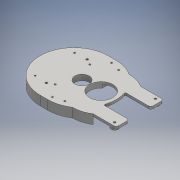
# Autodesk Inventor part: AZ-FLDIC-FWup top adapter
Saved by Autodesk Inventor 2016 (Build 200138000, 138)
## iProperties
Created: 2015-08-14
Part Number: AZ-FLDIC-FWup top adapter
Material: Generic
Document SubType Name: Modeling
Designer: kthorn
Density: 1 g/cm^3
Appearance: Default
Author: kthorn
Autodesk Inventor part; units mm, degrees
ref_plane "YZ Plane" through (0, 0, 0) normal (1, 0, 0) x (0, 1, 0)
ref_plane "XZ Plane" through (0, 0, 0) normal (0, 1, 0) x (-1, 0, 0)
ref_plane "XY Plane" through (0, 0, 0) normal (0, 0, 1) x (1, 0, 0)
sketch "Sketch1" plane through (0, 0, 0) normal (0, 0, 1) x (1, 0, 0)
  line L0 (-19.2849, 35) -> (-19.2849, -35) construction
  line L1 (19.7114, 54.5) -> (19.7114, -54.5) construction
  line L2 (-19.2849, 35) -> (19.7114, 54.5) construction
  line L3 (-19.2849, -35) -> (19.7114, -54.5) construction
  circle A0 centre (0.08, 0) radius 14.5
  line L4 (-19.2849, 35) -> (0.08, 0) construction
  line L5 (0.08, 0) -> (-19.2849, -35) construction
  circle A1 centre (19.7114, 54.5) radius 1.75
  circle A2 centre (-19.2849, 35) radius 1.75
  circle A3 centre (-19.2849, -35) radius 1.75
  circle A4 centre (19.7114, -54.5) radius 1.75
  line L6 (-16, -69) -> (0, -69)
  line L7 (0, 69) -> (-16, 69)
  arc A5 (-16, 69) -> (-16, -69) centre (-16, 0) ccw
  arc A6 (0, -69) -> (0, 69) centre (0, 0) ccw
  line L8 (-85, 0) -> (69, 0) construction
  circle A7 centre (-19.2849, 35) radius 3
  circle A8 centre (-19.2849, -35) radius 3
  circle A9 centre (19.7114, 54.5) radius 3
  circle A10 centre (19.7114, -54.5) radius 3
  line L9 (0, -60) -> (0, 60) construction
  line L10 (-55, 40) -> (-55, -40) construction
  circle A11 centre (-55, 40) radius 1.65
  circle A12 centre (-55, -40) radius 1.65
  circle A13 centre (0, -60) radius 1.65
  circle A14 centre (0, 60) radius 1.65
  point P0 (-19.2849, 0)
  point P1 (19.7114, 0)
  point P2 (-55, 0)
  dimension "d0" = 70
  dimension "d1" = 109
  dimension "d2" = 43.6
  dimension "d3" = 29
  dimension "d4" = 40
  dimension "d5" = 3.5
  dimension "d7" = 138
  dimension "d8" = 154
  dimension "d33" = 6
  dimension "d55" = 85.08
  dimension "d110" = 120
  dimension "d111" = 30
  dimension "d112" = 80
  dimension "d113" = 3.3
  constraints: 22 end point, 15 centre point, 14 coincident, 9 equal radius, 6 point on circle, 4 midpoint, 4 vertical, 3 equal length, 3 point on line, 2 tangent, 1 horizontal, 1 parallel
  measures "d0" distance of L0.start L0.end
  measures "d1" distance of L1.start L1.end
  measures "d2" distance of L0.start L1.start
  measures "d3" diameter of A0
  measures "d4" distance of L0.start L4.end
  measures "d5" diameter of A1
  measures "d7" distance of L7.end L6.start
  measures "d8" distance of L8.start L8.end
  measures "d33" diameter of A8
  measures "d55" distance of L4.end L8.start
  measures "d110" distance of L9.start L9.end
  measures "d111" distance from line of L8.start L10
  measures "d112" distance of L10.start L10.end
  measures "d113" diameter of A11
extrude "Extrusion1" add sketch "Sketch1" along normal blind 19 contours A5 L7 A6 L6 | A7 | A8 | A9 | A10 | A11 | A12 | A13 | A14
sketch "Sketch2" plane through (0, 0, 19) normal (0, 0, 1) x (1, 0, 0)
  circle A0 centre (-52.47, 0) radius 18.5329 construction
  circle A1 centre (-71.0029, 0) radius 2
  circle A2 centre (-43.2035, 16.05) radius 2
  circle A3 centre (-43.2035, -16.05) radius 2
  circle A4 centre (0.08, 0) radius 14.5 projected
  circle A5 centre (19.7114, -54.5) radius 1.75 projected
  circle A6 centre (-19.2849, -35) radius 1.75 projected
  circle A7 centre (-19.2849, 35) radius 1.75 projected
  circle A8 centre (19.7114, 54.5) radius 1.75 projected
  line L0 (-16, -69) -> (0, -69) projected
  arc A9 (0, -69) -> (0, 69) centre (0, 0) ccw projected
  line L1 (0, 69) -> (-16, 69) projected
  arc A10 (-16, 69) -> (-16, -69) centre (-16, 0) ccw projected
  arc A11 (-16, 69) -> (-16, -69) centre (-16, 0) ccw construction
  line L2 (-85, 0) -> (69, 0) construction
  circle A12 centre (-43.2035, -16.05) radius 5
  circle A13 centre (-43.2035, 16.05) radius 5
  circle A14 centre (-71.0029, 0) radius 5
  dimension "d11" = 120
  dimension "d12" = 120
  dimension "d13" = 32.1
  dimension "d14" = 52.55
  dimension "d40" = 4
  dimension "d49" = 10
  constraints: 7 centre point, 6 point on circle, 4 equal radius, 3 coincident, 2 end point, 2 point on line
  measures "d13" distance of A2.centre A1.centre
  measures "d14" distance of A0.centre A4.centre
  measures "d40" diameter of A2
  measures "d49" diameter of A13
sketch "Sketch3" plane through (0, 0, 0) normal (0, 0, -1) x (-1, 0, 0)
  circle A0 centre (30.8533, 41.3) radius 2.1
  circle A1 centre (-0.08, 0) radius 14.5 projected
  circle A2 centre (30.8533, -41.3) radius 2.1
  line L0 (30.8533, 41.3) -> (-0.08, 0) construction
  line L1 (-0.08, 0) -> (30.8533, -41.3) construction
  circle A3 centre (-0.08, 0) radius 14.5 construction
  circle A4 centre (-19.7114, -54.5) radius 1.75 construction
  circle A5 centre (19.2849, -35) radius 1.75 construction
  circle A6 centre (19.2849, 35) radius 1.75 construction
  circle A7 centre (-19.7114, 54.5) radius 1.75 construction
  line L2 (16, -69) -> (0, -69) construction
  arc A8 (16, -69) -> (16, 69) centre (16, 0) ccw construction
  line L3 (0, 69) -> (16, 69) construction
  arc A9 (0, 69) -> (0, -69) centre (0, 0) ccw construction
  arc A10 (16, -69) -> (16, 69) centre (16, 0) ccw construction
  line L4 (85, 0) -> (-69, 0) construction
  arc A11 (0, 69) -> (0, -69) centre (0, 0) ccw construction
  line L5 (30.8533, 41.3) -> (30.8533, -41.3)
  line L6 (37.5533, 48) -> (-142.6467, 48)
  line L7 (-142.6467, 48) -> (-142.6467, -48)
  line L8 (-142.6467, -48) -> (37.5533, -48)
  line L9 (37.5533, -48) -> (37.5533, 48)
  line L10 (30.8533, 41.3) -> (37.5533, 41.3) construction
  line L11 (30.8533, 41.3) -> (30.8533, 48) construction
  line L12 (30.8533, -41.3) -> (37.5533, -41.3) construction
  line L13 (30.8533, -41.3) -> (30.8533, -48) construction
  circle A12 centre (-107.4467, 41.3) radius 2.1
  circle A13 centre (-107.4467, -41.3) radius 2.1
  line L14 (30.8533, 41.3) -> (-107.4467, 41.3) construction
  line L15 (30.8533, -41.3) -> (-107.4467, -41.3) construction
  line L16 (-23.4467, 48) -> (-23.4467, -48)
  circle A14 centre (-38.88, 0) radius 23.5
  circle A15 centre (-38.88, 0) radius 55.5
  arc A16 (-38.1482, 57.4953) -> (-70.5383, 48) centre (-38.88, 0) ccw
  arc A17 (-70.5383, -48) -> (-38.1482, -57.4953) centre (-38.88, 0) ccw
  line L17 (-38.1482, 57.4953) -> (-38.1482, 48)
  line L18 (-70.5383, 48) -> (-38.1482, 48)
  line L19 (-38.1482, -57.4953) -> (-38.1482, -48)
  line L20 (-70.5383, -48) -> (-38.1482, -48)
  dimension "d15" = 51.6
  dimension "d18" = 82.6
  dimension "d20" = 180.2
  dimension "d22" = 96
  dimension "d29" = 138.3
  dimension "d59" = 4.2
  dimension "d61" = 61
  dimension "d68" = 47
  dimension "d69" = 38.8
  dimension "d70" = 69
  dimension "d118" = 111
  dimension "d141" = 2
  constraints: 38 end point, 12 point on line, 10 point on circle, 8 centre point, 7 perpendicular, 4 equal length, 3 coincident, 3 equal radius, 3 horizontal, 3 parallel, 1 collinear, 1 vertical
  measures "d15" distance of L0.end L0.start
  measures "d18" distance of L0.start L1.end
  measures "d20" distance of L7.end L8.end
  measures "d22" distance of L6.end L7.end
  measures "d29" distance of L1.end L15.end
  measures "d59" diameter of A13
  measures "d61" distance between parallel lines of L16 L9
  measures "d68" diameter of A14
  measures "d69" distance of A14.centre L0.end
  measures "d70" distance from line of A14.centre L2
  measures "d118" diameter of A15
  measures "d141" radial gap between concentric circles of A15 A17
extrude "Extrusion14" cut sketch "Sketch3" against normal blind 14 contours L16 A14 L8 A15 L6 | L16 A14 | A15 L8 L7 L6 picked at (-49.8352, 39.5964) picked at (-36.3678, -0.9407)
extrude "Extrusion15" cut sketch "Sketch3" against normal blind 7.5 contours L6 A15 L8 L16 A14 | L6 L9 L8 A15 | A14 L16 picked at (-10.5973, 24.5754) picked at (-22.3115, -4.6826)
extrude "Extrusion16" cut sketch "Sketch3" against normal through all contours A0 | A2
sketch "Sketch8" plane through (0, 0, 19) normal (0, 0, 1) x (1, 0, 0)
  line L0 (-37.5533, 48) -> (-37.5533, -48) projected
  circle A0 centre (107.4467, -41.3) radius 2.1 projected
  circle A1 centre (107.4467, 41.3) radius 2.1 projected
  line L1 (-37.5533, -48) -> (117.4467, -48)
  line L2 (117.4467, -48) -> (117.4467, -22)
  line L3 (117.4467, -22) -> (-37.5533, -22)
  line L4 (-37.5533, -22) -> (-37.5533, -48)
  line L5 (49.5681, 48) -> (-37.5533, 48) projected
  line L6 (-37.5533, 48) -> (117.4467, 48)
  line L7 (117.4467, 48) -> (117.4467, 22)
  line L8 (117.4467, 22) -> (-37.5533, 22)
  line L9 (-37.5533, 22) -> (-37.5533, 48)
  circle A2 centre (107.4467, -41.3) radius 2.1
  circle A3 centre (107.4467, 41.3) radius 2.1
  arc A4 (109.474, -48) -> (105.4194, -48) centre (107.4467, -41.3) ccw
  arc A5 (105.4194, 48) -> (109.474, 48) centre (107.4467, 41.3) ccw
  point P0 (122.0315, -50.7282)
  point P1 (122.0315, 31.8718)
  dimension "d79" = 26
  dimension "d80" = 155
  dimension "d81" = 14
  constraints: 16 end point, 5 point on line, 4 centre point, 4 coincident, 4 parallel, 4 point on circle, 3 equal radius, 2 horizontal, 2 perpendicular, 1 collinear
  measures "d79" distance of L6.end L7.end
  measures "d80" distance of L0.end L1.end
  measures "d81" diameter of A4
extrude "Extrusion18" add sketch "Sketch8" against normal up to surface (5 mm away)
extrude "Extrusion19" add sketch "Sketch8" against normal blind 9 contours L6 A5 | A4 L1
extrude "Extrusion17" cut sketch "Sketch3" against normal through all contours A14 L16 | L16 A14
extrude "Extrusion20" cut sketch "Sketch3" against normal through all contours A0 | A2
extrude "Extrusion21" cut sketch "Sketch1" along normal through all contours A2 | A3
extrude "Extrusion22" cut sketch "Sketch1" along normal blind 14 contours A7 | A8 | A9 | A10
extrude "Extrusion23" cut sketch "Sketch1" along normal through all contours A11 | A12 | A13 | A14
fillet "Fillet1" radius 5 1 edges at (117.4467, 48, 16.5)
fillet "Fillet2" radius 5 3 edges at (117.4467, 22, 16.5) (117.4467, -22, 16.5) (117.4467, -48, 16.5)
thread "Thread1" size "M5x0.8" class "6H" standard "ANSI Metric M Profile" full length
thread "Thread2" size "M5x0.8" class "6H" standard "ANSI Metric M Profile" full length
thread "Thread3" size "M5x0.8" class "6H" standard "ANSI Metric M Profile" full length
thread "Thread4" size "M5x0.8" class "6H" standard "ANSI Metric M Profile" full length
thread "Thread6" size "M4x0.7" class "6H" standard "ANSI Metric M Profile" full length
thread "Thread7" size "M4x0.7" class "6H" standard "ANSI Metric M Profile" full length
thread "Thread8" size "M4x0.7" class "6H" standard "ANSI Metric M Profile" full length
thread "Thread9" size "M4x0.7" class "6H" standard "ANSI Metric M Profile" full length
fillet "Fillet3" radius 2 2 edges at (65.3988, 22, 16.5) (65.3988, -22, 16.5)
extrude "Extrusion27" add sketch "Sketch3" against normal up to surface (19 mm away) contours L6 A15 L17 | L6 A16 L17 A15 | A15 L19 A17 L8 | L8 L19 A15 picked at (-54.2009, 49.4023) picked at (-54.2009, -49.4023)
extrude "Extrusion26" cut sketch "Sketch3" against normal blind 4 contours L16 A14 L8 A15 L6 | L6 L17 A15 | L6 A15 L8 L16 A14 | L6 A15 L17 | L8 L19 A15 | A15 L19 L8
chamfer "Chamfer2" distance 1 angle 45 4 edges at (22.2868, 52.9615, 2) (18.6661, 51.688, 2) (18.6661, -51.688, 2) (22.2868, -52.9615, 2)
sketch "Sketch10" plane through (0, 0, 7.5) normal (0, 0, -1) x (-1, 0, 0)
  line L0 (37.5533, 48) -> (37.5533, -48) projected
  line L1 (37.5533, 48) -> (22.5533, 48)
  line L2 (22.5533, 48) -> (22.5533, 34.5)
  line L3 (22.5533, 34.5) -> (37.5533, 34.5)
  line L4 (37.5533, 34.5) -> (37.5533, 48)
  line L5 (37.5533, -48) -> (22.5533, -48)
  line L6 (22.5533, -48) -> (22.5533, -34.5)
  line L7 (22.5533, -34.5) -> (37.5533, -34.5)
  line L8 (37.5533, -34.5) -> (37.5533, -48)
  point P0 (0, 0)
  dimension "d149" = 13.5
  dimension "d150" = 15
  constraints: 16 end point, 4 parallel, 2 horizontal, 2 perpendicular, 1 collinear, 1 point on line
  measures "d149" distance of L1.end L2.end
  measures "d150" distance of L2.end L3.end
extrude "Extrusion29" cut sketch "Sketch10" against normal blind 1.2
body "Solid1"
